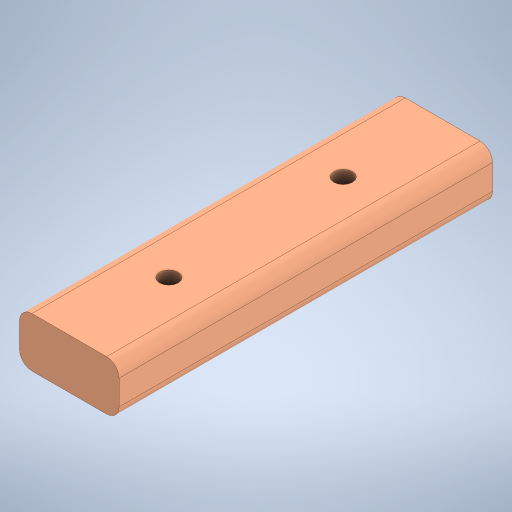
# Autodesk Inventor part: Wood-1
Saved by Autodesk Inventor 2024 (Build 280153000, 153)
## iProperties
Created: 2024-03-20
Part Number: Wood-1
Material: Generic
Document SubType Name: Modeling
Designer: Liz
Density: 1 g/cm^3
Appearance: Default
Author: Liz
Autodesk Inventor part; units mm, degrees
ref_plane "YZ Plane" through (0, 0, 0) normal (1, 0, 0) x (0, 1, 0)
ref_plane "XZ Plane" through (0, 0, 0) normal (0, 1, 0) x (-1, 0, 0)
ref_plane "XY Plane" through (0, 0, 0) normal (0, 0, 1) x (1, 0, 0)
sketch "Sketch1" plane through (0, 0, 0) normal (0, 0, 1) x (1, 0, 0)
  line L0 (-38.1, -25.4) -> (38.1, -25.4)
  line L1 (50.8, -12.7) -> (50.8, 12.7)
  line L2 (38.1, 25.4) -> (-38.1, 25.4)
  line L3 (-50.8, 12.7) -> (-50.8, -12.7)
  line L4 (-50.8, -25.4) -> (50.8, 25.4) construction
  line L5 (50.8, -25.4) -> (-50.8, 25.4) construction
  arc A0 (-38.1, 25.4) -> (-50.8, 12.7) centre (-38.1, 12.7) ccw
  arc A1 (-50.8, -12.7) -> (-38.1, -25.4) centre (-38.1, -12.7) ccw
  arc A2 (38.1, -25.4) -> (50.8, -12.7) centre (38.1, -12.7) ccw
  arc A3 (50.8, 12.7) -> (38.1, 25.4) centre (38.1, 12.7) ccw
  point P0 (0, 0)
  dimension "d0" = 12.7
  dimension "d1" = 101.6
  dimension "d2" = 50.8
  constraints: 12 end point, 8 point on circle, 8 point on line, 8 tangent, 4 centre point, 3 equal radius, 2 midpoint, 2 parallel, 1 horizontal, 1 perpendicular
  measures "d0" radius of A0
  measures "d1" distance between parallel lines of L1 L3
  measures "d2" distance between parallel lines of L0 L2
extrude "Extrusion1" add sketch "Sketch1" along normal blind 381
sketch "Sketch2" plane through (-38.1, 25.4, 0) normal (0, 1, 0) x (1, 0, 0)
  circle A0 centre (38.1, -279.4) radius 9.525
  circle A1 centre (38.1, -101.6) radius 9.525
  line L0 (-12.7, 0) -> (-12.7, -381) projected
  line L1 (76.2, 0) -> (0, 0) projected
  point P0 (38.1, 0)
  point P1 (-12.7, -190.5)
  point P2 (38.1, 0)
  dimension "d6" = 88.9
  dimension "d7" = 19.05
  dimension "d8" = 177.8
  constraints: 2 centre point, 2 midpoint, 2 vertical alignment, 1 equal radius
  measures "d6" vertical distance of point (-12.7, -190.5) A0.centre
  measures "d7" diameter of A0
  measures "d8" distance of A1.centre A0.centre
extrude "Extrusion2" cut sketch "Sketch2" against normal blind 381
body "Solid1"
